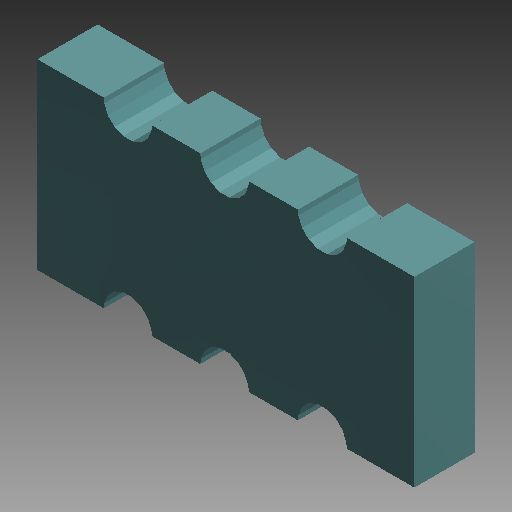
# Autodesk Inventor part: 1K
Saved by Autodesk Inventor 2018.2 (Build 222227000, 227)
## iProperties
Part Number: 1K
Material: Generic
Document SubType Name: Modeling
Designer: autocad
Appearance: CAY16, 1K
Author: autocad
Autodesk Inventor part; units mm, degrees
ref_plane "YZ Plane" through (0, 0, 0) normal (1, 0, 0) x (0, 1, 0)
ref_plane "XZ Plane" through (0, 0, 0) normal (0, 1, 0) x (-1, 0, 0)
ref_plane "XY Plane" through (0, 0, 0) normal (0, 0, 1) x (1, 0, 0)
sketch "CAY16, 1K_278" plane through (0, 0, 0) normal (0, 0, 1) x (1, 0, 0)
  line L0 (-1.5505, 0.7625) -> (-0.9999, 0.7625)
  line L1 (-0.9999, 0.7625) -> (-0.9997, 0.7624)
  line L2 (-0.9997, 0.7624) -> (-0.9996, 0.7623)
  line L3 (-0.9996, 0.7623) -> (-0.9995, 0.7621)
  line L4 (-0.9995, 0.7621) -> (-0.9995, 0.762)
  line L5 (-0.9995, 0.762) -> (-0.9957, 0.7231)
  line L6 (-0.9957, 0.7231) -> (-0.9659, 0.6512)
  line L7 (-0.9659, 0.6512) -> (-0.9108, 0.5961)
  line L8 (-0.9108, 0.5961) -> (-0.8389, 0.5663)
  line L9 (-0.8389, 0.5663) -> (-0.7611, 0.5663)
  line L10 (-0.7611, 0.5663) -> (-0.6892, 0.5961)
  line L11 (-0.6892, 0.5961) -> (-0.6341, 0.6512)
  line L12 (-0.6341, 0.6512) -> (-0.6043, 0.7231)
  line L13 (-0.6043, 0.7231) -> (-0.6005, 0.762)
  line L14 (-0.6005, 0.762) -> (-0.6005, 0.7621)
  line L15 (-0.6005, 0.7621) -> (-0.6004, 0.7623)
  line L16 (-0.6004, 0.7623) -> (-0.6003, 0.7624)
  line L17 (-0.6003, 0.7624) -> (-0.6001, 0.7625)
  line L18 (-0.6001, 0.7625) -> (-0.1999, 0.7625)
  line L19 (-0.1999, 0.7625) -> (-0.1997, 0.7624)
  line L20 (-0.1997, 0.7624) -> (-0.1996, 0.7623)
  line L21 (-0.1996, 0.7623) -> (-0.1995, 0.7621)
  line L22 (-0.1995, 0.7621) -> (-0.1995, 0.762)
  line L23 (-0.1995, 0.762) -> (-0.1956, 0.7228)
  line L24 (-0.1956, 0.7228) -> (-0.1656, 0.6503)
  line L25 (-0.1656, 0.6503) -> (-0.1101, 0.5948)
  line L26 (-0.1101, 0.5948) -> (-0.0376, 0.5648)
  line L27 (-0.0376, 0.5648) -> (0.0408, 0.5648)
  line L28 (0.0408, 0.5648) -> (0.1133, 0.5948)
  line L29 (0.1133, 0.5948) -> (0.1688, 0.6503)
  line L30 (0.1688, 0.6503) -> (0.1988, 0.7228)
  line L31 (0.1988, 0.7228) -> (0.2027, 0.762)
  line L32 (0.2027, 0.762) -> (0.2027, 0.7621)
  line L33 (0.2027, 0.7621) -> (0.2028, 0.7623)
  line L34 (0.2028, 0.7623) -> (0.2029, 0.7624)
  line L35 (0.2029, 0.7624) -> (0.2031, 0.7625)
  line L36 (0.2031, 0.7625) -> (0.6097, 0.7625)
  line L37 (0.6097, 0.7625) -> (0.6099, 0.7624)
  line L38 (0.6099, 0.7624) -> (0.61, 0.7623)
  line L39 (0.61, 0.7623) -> (0.6101, 0.7621)
  line L40 (0.6101, 0.7621) -> (0.6101, 0.762)
  line L41 (0.6101, 0.762) -> (0.614, 0.7225)
  line L42 (0.614, 0.7225) -> (0.6443, 0.6494)
  line L43 (0.6443, 0.6494) -> (0.7002, 0.5935)
  line L44 (0.7002, 0.5935) -> (0.7733, 0.5632)
  line L45 (0.7733, 0.5632) -> (0.8523, 0.5632)
  line L46 (0.8523, 0.5632) -> (0.9254, 0.5935)
  line L47 (0.9254, 0.5935) -> (0.9814, 0.6494)
  line L48 (0.9814, 0.6494) -> (1.0116, 0.7225)
  line L49 (1.0116, 0.7225) -> (1.0155, 0.762)
  line L50 (1.0155, 0.762) -> (1.0155, 0.7621)
  line L51 (1.0155, 0.7621) -> (1.0156, 0.7623)
  line L52 (1.0156, 0.7623) -> (1.0157, 0.7624)
  line L53 (1.0157, 0.7624) -> (1.0159, 0.7625)
  line L54 (1.0159, 0.7625) -> (1.5753, 0.7625)
  line L55 (1.5753, 0.7625) -> (1.5753, -0.7505)
  line L56 (1.5753, -0.7505) -> (1.0155, -0.7505)
  line L57 (1.0155, -0.7505) -> (1.0155, -0.75)
  line L58 (1.0155, -0.75) -> (1.0116, -0.7105)
  line L59 (1.0116, -0.7105) -> (0.9814, -0.6374)
  line L60 (0.9814, -0.6374) -> (0.9254, -0.5815)
  line L61 (0.9254, -0.5815) -> (0.8523, -0.5512)
  line L62 (0.8523, -0.5512) -> (0.7733, -0.5512)
  line L63 (0.7733, -0.5512) -> (0.7002, -0.5815)
  line L64 (0.7002, -0.5815) -> (0.6443, -0.6374)
  line L65 (0.6443, -0.6374) -> (0.614, -0.7105)
  line L66 (0.614, -0.7105) -> (0.6101, -0.75)
  line L67 (0.6101, -0.75) -> (0.6101, -0.7501)
  line L68 (0.6101, -0.7501) -> (0.61, -0.7503)
  line L69 (0.61, -0.7503) -> (0.6099, -0.7504)
  line L70 (0.6099, -0.7504) -> (0.6097, -0.7505)
  line L71 (0.6097, -0.7505) -> (0.2027, -0.7505)
  line L72 (0.2027, -0.7505) -> (0.2027, -0.75)
  line L73 (0.2027, -0.75) -> (0.1988, -0.7108)
  line L74 (0.1988, -0.7108) -> (0.1688, -0.6383)
  line L75 (0.1688, -0.6383) -> (0.1133, -0.5828)
  line L76 (0.1133, -0.5828) -> (0.0408, -0.5528)
  line L77 (0.0408, -0.5528) -> (-0.0376, -0.5528)
  line L78 (-0.0376, -0.5528) -> (-0.1101, -0.5828)
  line L79 (-0.1101, -0.5828) -> (-0.1656, -0.6383)
  line L80 (-0.1656, -0.6383) -> (-0.1956, -0.7108)
  line L81 (-0.1956, -0.7108) -> (-0.1995, -0.75)
  line L82 (-0.1995, -0.75) -> (-0.1995, -0.7501)
  line L83 (-0.1995, -0.7501) -> (-0.1996, -0.7503)
  line L84 (-0.1996, -0.7503) -> (-0.1997, -0.7504)
  line L85 (-0.1997, -0.7504) -> (-0.1999, -0.7505)
  line L86 (-0.1999, -0.7505) -> (-0.6005, -0.7505)
  line L87 (-0.6005, -0.7505) -> (-0.6005, -0.75)
  line L88 (-0.6005, -0.75) -> (-0.6043, -0.7111)
  line L89 (-0.6043, -0.7111) -> (-0.6341, -0.6392)
  line L90 (-0.6341, -0.6392) -> (-0.6892, -0.5841)
  line L91 (-0.6892, -0.5841) -> (-0.7611, -0.5544)
  line L92 (-0.7611, -0.5544) -> (-0.8389, -0.5544)
  line L93 (-0.8389, -0.5544) -> (-0.9108, -0.5841)
  line L94 (-0.9108, -0.5841) -> (-0.9659, -0.6392)
  line L95 (-0.9659, -0.6392) -> (-0.9957, -0.7111)
  line L96 (-0.9957, -0.7111) -> (-0.9995, -0.75)
  line L97 (-0.9995, -0.75) -> (-0.9995, -0.7501)
  line L98 (-0.9995, -0.7501) -> (-0.9996, -0.7503)
  line L99 (-0.9996, -0.7503) -> (-0.9997, -0.7504)
  line L100 (-0.9997, -0.7504) -> (-0.9999, -0.7505)
  line L101 (-0.9999, -0.7505) -> (-1.5505, -0.7505)
  line L102 (-1.5505, -0.7505) -> (-1.5505, 0.7625)
  constraints: 206 end point
extrude "Extrusion1" add sketch "CAY16, 1K_278" along normal blind 0.5
body "Solid1"
